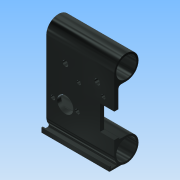
# Autodesk Inventor part: каретка  хотэнда
Saved by Autodesk Inventor 2017 (Build 210142000, 142)
## iProperties
Part Number: каретка  хотэнда
Material: Типовые
Document SubType Name: Modeling
Designer: Max
Mass: 13.8146 g
Surface Area: 148.178 cm^2
Volume: 13.8146 cm^3
Density: 1 g/cm^3
Appearance: Оружейный металл — полированный
Author: Max
Autodesk Inventor part; units mm, degrees
ref_plane "YZ Plane" through (0, 0, 0) normal (1, 0, 0) x (0, 1, 0)
ref_plane "XZ Plane" through (0, 0, 0) normal (0, 1, 0) x (-1, 0, 0)
ref_plane "XY Plane" through (0, 0, 0) normal (0, 0, 1) x (1, 0, 0)
sketch "Эскиз1" plane through (0, 0, 0) normal (1, 0, 0) x (0, 1, 0)
  line L0 (0, 0) -> (143.27187, 0) construction
  line L1 (0, 0) -> (0, -170.504512) construction
  arc A0 (0, -8.91) -> (-8.91, 0) centre (0, 0) ccw
  circle A1 centre (0, -52.3) radius 7.5
  circle A2 centre (0, 0) radius 7.5
  line L2 (-8.91, 0) -> (-8.91, -52.3)
  line L3 (-5.91, -10.91) -> (-5.91, -41.39)
  line L4 (0, -8.91) -> (-3.91, -8.91)
  line L5 (0, -43.39) -> (-3.91, -43.39)
  line L6 (-12.45, -60.45) -> (-12.45, -57.11)
  line L7 (-12.45, -57.11) -> (-11.45, -57.11)
  line L8 (-11.45, -57.11) -> (-11.45, -59.11)
  line L9 (-11.45, -59.11) -> (-8.0282, -59.11)
  arc A3 (-8.91, -52.3) -> (-7.218089, -57.523724) centre (0, -52.3) ccw
  arc A4 (-3.267299, -60.589322) -> (0, -43.39) centre (0, -52.3) ccw
  circle A5 centre (0, 0) radius 4 construction
  line L10 (0, 4) -> (-17.853128, 4) construction
  line L11 (-17.853128, 4) -> (-17.853128, -60.45) construction
  line L12 (-17.853128, -60.45) -> (-12.45, -60.45) construction
  line L13 (-12.45, -60.45) -> (-4.0007, -60.45)
  arc A6 (-8.0282, -59.11) -> (-7.218089, -57.523724) centre (-8.0282, -58.11) ccw
  arc A7 (-5.91, -41.39) -> (-3.91, -43.39) centre (-3.91, -41.39) ccw
  arc A8 (-3.91, -8.91) -> (-5.91, -10.91) centre (-3.91, -10.91) ccw
  arc A9 (-3.267299, -60.589322) -> (-4.0007, -60.45) centre (-4.0007, -62.45) ccw
  point P0 (-5.91, -43.39)
  point P1 (-5.91, -8.91)
  point P2 (0, -61.21)
  point P3 (-5.745607, -59.11)
  point P4 (-3.600778, -60.45)
  dimension "d34" = 8
  dimension "d0" = 17.82
  dimension "d2" = 15
  dimension "d3" = 15
  dimension "d4" = 52.3
  dimension "d5" = 3
  dimension "d9" = 1
  dimension "d11" = 8.91
  dimension "d12" = 8.91
  dimension "d13" = 3.54
  dimension "d35" = 64.45
  dimension "d36" = 3.34
  dimension "d37" = 1.34
  dimension "d38" = 1
  dimension "d39" = 2
  dimension "d40" = 2
  dimension "d41" = 2
  dimension "d42" = 63.11
  dimension "d43" = 70.12
  constraints: 28 end point, 17 point on circle, 12 tangent, 10 point on line, 9 centre point, 5 perpendicular, 4 coincident, 3 horizontal, 2 parallel, 1 collinear, 1 vertical, 1 vertical alignment, 2 other
  measures "d0" diameter of A0
  measures "d2" diameter of A1
  measures "d3" diameter of A2
  measures "d4" distance of L0.start A3.centre
  measures "d5" distance between parallel lines of L2 L3
  measures "d9" distance between parallel lines of L6 L8
  measures "d11" radius of A4
  measures "d12" radius of A3
  measures "d13" distance from line of L6 L2.end
  measures "d35" distance of L10.end L11.end
  measures "d36" distance between parallel lines of L7 L13
  measures "d37" distance between parallel lines of L13 L9
  measures "d38" radius of A6
  measures "d39" radius of A7
  measures "d40" radius of A8
  measures "d41" radius of A9
  measures "d42" distance from line of L10.start L9
extrude "Выдавливание1" add sketch "Эскиз1" along normal mid plane 50
sketch "Эскиз2" plane through (-25, -5.91, -8.91) normal (0, 1, 0) x (1, 0, 0)
  circle A0 centre (13.95, 28.46) radius 5.95
  line L0 (4.95, 28.46) -> (13.95, 28.46) construction
  line L1 (13.95, 28.46) -> (24.436318, 28.46) construction
  circle A1 centre (4.95, 28.46) radius 1.6
  circle A2 centre (22.95, 28.46) radius 1.6
  line L2 (13.95, 28.46) -> (13.95, 32.27883)
  circle A3 centre (4.95, 28.46) radius 1.455 construction
  circle A4 centre (22.95, 28.46) radius 1.455 construction
  line L3 (0, 5.642815) -> (0, 38.122815) construction
  line L4 (50, -8.91) -> (50, 43.39) construction
  line L5 (50, 14.93) -> (39.51, 14.93)
  line L6 (39.51, 14.93) -> (39.51, 33.09)
  line L7 (39.51, 33.09) -> (50, 33.09)
  line L8 (50, 33.09) -> (50, 14.93)
  line L9 (0, -18.82) -> (50, -18.82) construction
  line L10 (50, 43.39) -> (2.383382, 43.39)
  line L11 (50, -17.82) -> (50, 0)
  line L12 (50, -17.82) -> (50, 0)
  line L13 (50, -8.91) -> (53.294914, -8.91)
  line L14 (50, -12.91) -> (54.162489, -12.91)
  line L15 (0, 52.3) -> (50, 52.3)
  dimension "d15" = 3.2
  dimension "d16" = 3.2
  dimension "d17" = 2.91
  dimension "d18" = 2.91
  dimension "d21" = 18
  dimension "d22" = 11.9
  dimension "d23" = 8
  dimension "d25" = 39.51
  dimension "d27" = 18.16
  dimension "d44" = 17.82
  dimension "d45" = 8.91
  dimension "d46" = 8.91
  dimension "d48" = 4
  dimension "d49" = 46
  dimension "d50" = 10.49
  dimension "d51" = 19.61
  dimension "d52" = 17.89
  constraints: 28 end point, 5 centre point, 4 horizontal, 4 point on line, 3 coincident, 3 equal length, 2 collinear, 1 perpendicular, 1 symmetric about line, 1 vertical
  measures "d15" diameter of A1
  measures "d16" diameter of A2
  measures "d17" diameter of A3
  measures "d18" diameter of A4
  measures "d21" distance of A2.centre L0.start
  measures "d22" diameter of A0
  measures "d23" distance edge to line of A0 L3
  measures "d25" distance between parallel lines of L6 L3
  measures "d27" distance between parallel lines of L7 L5
  measures "d44" distance of L11.start L11.end
  measures "d45" distance from line of L13 L11.end
  measures "d46" distance from line of L13 L11.start
  measures "d48" distance between parallel lines of L13 L14
  measures "d49" distance between parallel lines of L7 L14
  measures "d50" distance between parallel lines of L4 L6
  measures "d51" distance edge to line of A0 L6
  measures "d52" distance edge to line of A0 L15
extrude "Выдавливание2" cut sketch "Эскиз2" along normal mid plane 50
sketch "Эскиз4" plane through (-25, -5.91, -10.91) normal (0, 1, 0) x (1, 0, 0)
  line L0 (14.05, 0.23) -> (37.55, 0.23) construction
  circle A0 centre (14.05, 0.23) radius 2.05
  circle A1 centre (37.55, 0.23) radius 2.05
  line L1 (0, -19.82) -> (50, -19.82) construction
  line L2 (0, 0) -> (0, 30.48) construction
  line L3 (50, 12.93) -> (50, 0) projected
  point P0 (25, -10.91)
  dimension "d53" = 4.1
  dimension "d54" = 4.1
  dimension "d57" = 18
  dimension "d61" = 19.4
  dimension "d63" = 14.05
  dimension "d65" = 23.5
  constraints: 2 centre point, 2 coincident, 2 end point, 1 horizontal
  measures "d53" diameter of A0
  measures "d54" diameter of A1
  measures "d57" distance edge to line of A0 L1
  measures "d63" distance from line of L2 L0.start
  measures "d65" distance of L0.end L0.start
extrude "Выдавливание3" cut sketch "Эскиз4" along normal mid plane 50
sketch "Эскиз6" plane through (-25, -5.91, -10.91) normal (0, 1, 0) x (1, 0, 0)
  circle A0 centre (42, 7.46) radius 1.5
  arc A1 (16.087057, 0) -> (12.012943, 0) centre (14.05, 0.23) ccw
  circle A2 centre (14.05, 0.23) radius 2
  arc A3 (39.587057, 0) -> (35.512943, 0) centre (37.55, 0.23) ccw
  circle A4 centre (37.55, 0.23) radius 2
  circle A5 centre (24, 7.46) radius 1.5
  circle A6 centre (4.95, 26.46) radius 1.129269
  spline S0 degree 3 poles (21.799899, 26.563204) (21.753431, 26.045363) (22.103055, 25.518519) (22.59827, 25.36015) (23.093485, 25.201782) (23.683934, 25.427991) (23.946568, 25.876703) (24.209201, 26.325414) (24.117313, 26.951) (23.73674, 27.305235) (23.356167, 27.659471) (22.725608, 27.706335) (22.296851, 27.41225) (21.868094, 27.118165) (21.684738, 26.513036) (21.878155, 26.03043) (22.071571, 25.547824) (22.622094, 25.236816) (23.135279, 25.320239) (23.648464, 25.403662) (24.072128, 25.873034) (24.102721, 26.392055) (24.133314, 26.911075) (23.767725, 27.426968) (23.267894, 27.570102) (22.768063, 27.713236) (22.184816, 27.469056) (21.936042, 27.012515) (21.687268, 26.555973) (21.798265, 25.933494) (22.189505, 25.591075) (22.580744, 25.248657) (23.212442, 25.221119) (23.631995, 25.528192) (24.051548, 25.835265) (24.216293, 26.445724) (24.008192, 26.922183) (23.800091, 27.398641) (23.240306, 27.692649) (22.729915, 27.593554) (22.219524, 27.494459) (21.810428, 27.012338) (21.795739, 26.492624) (21.78105, 25.972909) (22.162261, 25.468451) (22.66624, 25.340686) (23.170219, 25.212921) (23.745717, 25.474842) (23.980398, 25.938786) (24.215078, 26.40273) (24.085076, 27.021519) (23.683537, 27.3518) (23.281998, 27.68208) (22.649753, 27.690266) (22.239798, 27.370492) (21.829842, 27.050718) (21.683864, 26.435502) (21.906453, 25.965638) (22.129043, 25.495774) (22.697567, 25.219041) (23.204685, 25.333715) (23.711803, 25.448389) (24.105947, 25.942808) (24.104719, 26.462729) (24.10349, 26.982649) (23.707014, 27.475201) (23.199359, 27.587476) (22.691705, 27.699752) (22.124496, 27.420335) (21.904129, 26.949424) (21.683762, 26.478514) (21.832647, 25.863994) (22.244109, 25.546162) (22.655571, 25.228329) (23.28777, 25.239503) (23.687744, 25.571677) (24.087717, 25.903851) (24.214793, 26.523248) (23.977923, 26.986078) (23.741053, 27.448907) (23.164323, 27.708105) (22.660954, 27.57796) (22.157584, 27.447815) (21.778761, 26.94156) (21.795906, 26.421922) (21.813051, 25.902283) (22.224421, 25.4221) (22.735274, 25.325418) (23.246128, 25.228736) (23.804518, 25.525387) (24.010365, 26.002824) (24.216211, 26.48026) (24.048583, 27.089934) (23.627584, 27.39502) (23.206584, 27.700107) (22.575023, 27.669584) (22.185407, 27.325321) (21.79579, 26.981057) (21.687736, 26.35806) (21.938665, 25.9027) (22.189593, 25.447339) (22.773988, 25.205918) (23.273137, 25.351413) (23.772286, 25.496907) (24.135433, 26.014522) (24.102387, 26.533393) (24.069342, 27.052263) (23.643464, 27.519627) (23.12989, 27.600624) (22.616316, 27.681621) (22.06727, 27.368014) (21.876136, 26.8845) (21.685002, 26.400985) (21.871217, 25.796729) (22.301359, 25.504674) (22.731501, 25.212619) (23.361832, 25.262462) (23.740726, 25.618492) (24.119621, 25.974522) (24.208551, 26.600535) (23.9438, 27.048001) (23.679048, 27.495466) (23.087537, 27.718883) (22.593076, 27.558175) (22.098615, 27.397467) (21.751485, 26.868978) (21.8004, 26.351362) (21.849315, 25.833747) (22.289301, 25.37964) (22.805114, 25.314404) (23.320926, 25.249168) (23.860114, 25.579436) (24.036356, 26.068575) (24.212598, 26.557715) (24.007972, 27.155986) (23.56909, 27.434736) (23.130209, 27.713486) (22.5017, 27.644368) (22.133882, 27.276906) (21.961347, 27.104537) (21.845629, 26.876206) (21.808638, 26.635144) knots 2.61665571 2.61665571 2.61665571 2.61665571 3.96742673 3.96742673 3.96742673 5.31819776 5.31819776 5.31819776 6.66896878 6.66896878 6.66896878 8.01973981 8.01973981 8.01973981 9.37051084 9.37051084 9.37051084 10.72128186 10.72128186 10.72128186 12.07205289 12.07205289 12.07205289 13.42282392 13.42282392 13.42282392 14.77359494 14.77359494 14.77359494 16.12436597 16.12436597 16.12436597 17.475137 17.475137 17.475137 18.82590802 18.82590802 18.82590802 20.17667905 20.17667905 20.17667905 21.52745007 21.52745007 21.52745007 22.8782211 22.8782211 22.8782211 24.22899213 24.22899213 24.22899213 25.57976315 25.57976315 25.57976315 26.93053418 26.93053418 26.93053418 28.28130521 28.28130521 28.28130521 29.63207623 29.63207623 29.63207623 30.98284726 30.98284726 30.98284726 32.33361829 32.33361829 32.33361829 33.68438931 33.68438931 33.68438931 35.03516034 35.03516034 35.03516034 36.38593137 36.38593137 36.38593137 37.73670239 37.73670239 37.73670239 39.08747342 39.08747342 39.08747342 40.43824444 40.43824444 40.43824444 41.78901547 41.78901547 41.78901547 43.1397865 43.1397865 43.1397865 44.49055752 44.49055752 44.49055752 45.84132855 45.84132855 45.84132855 47.19209958 47.19209958 47.19209958 48.5428706 48.5428706 48.5428706 49.89364163 49.89364163 49.89364163 51.24441266 51.24441266 51.24441266 52.59518368 52.59518368 52.59518368 53.94595471 53.94595471 53.94595471 55.29672574 55.29672574 55.29672574 56.64749676 56.64749676 56.64749676 57.99826779 57.99826779 57.99826779 59.34903881 59.34903881 59.34903881 60.69980984 60.69980984 60.69980984 62.05058087 62.05058087 62.05058087 63.40135189 63.40135189 63.40135189 64.75212292 64.75212292 64.75212292 65.38573969 65.38573969 65.38573969 65.38573969
  circle A7 centre (22.95, 26.46) radius 1.6
  circle A8 centre (22.95, 26.46) radius 1.154622
  circle A9 centre (4.95, 26.46) radius 2.474109
  line L0 (-39.849119, 12.49) -> (304.043155, 12.49)
  line L1 (39.51, 31.09) -> (50, 31.09)
  line L2 (39.51, 12.93) -> (39.51, 30.48)
  line L3 (50, 12.93) -> (50, 0)
  point P0 (25, -10.91)
  dimension "d66" = 3
  dimension "d67" = 4
  dimension "d68" = 4
  dimension "d70" = 3
  dimension "d72" = 19
  dimension "d73" = 19
  dimension "d74" = 12.26
  dimension "d75" = 30.86
  dimension "d76" = 23.63
  dimension "d78" = 8
  dimension "d79" = 18
  constraints: 6 centre point, 4 coincident
  measures "d66" diameter of A0
  measures "d67" diameter of A2
  measures "d68" diameter of A4
  measures "d70" diameter of A5
  measures "d72" vertical distance of A0.centre A8.centre
  measures "d73" vertical distance of A8.centre A5.centre
  measures "d74" distance from line of L0 A4.centre
  measures "d75" distance from line of A4.centre L1
  measures "d76" distance from line of L1 A0.centre
  measures "d78" distance from line of L3 A0.centre
  measures "d79" distance of A0.centre A5.centre
extrude "Выдавливание4" cut sketch "Эскиз6" against normal blind 10 contours A0 | A5
